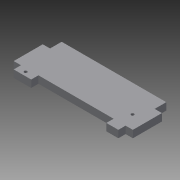
# Autodesk Inventor part: print-head-fix
Saved by Autodesk Inventor 2014 (Build 180170000, 170)
## iProperties
Created: 2014-03-01
Part Number: print-head-fix
Material: 常规
Document SubType Name: Modeling
Designer: Keshuai
Density: 1 g/cm^3
Appearance: 默认
Author: Keshuai
Autodesk Inventor part; units mm, degrees
ref_plane "YZ Plane" through (0, 0, 0) normal (1, 0, 0) x (0, 1, 0)
ref_plane "XZ Plane" through (0, 0, 0) normal (0, 1, 0) x (-1, 0, 0)
ref_plane "XY Plane" through (0, 0, 0) normal (0, 0, 1) x (1, 0, 0)
sketch "草图1" plane through (0, 0, 0) normal (0, 0, 1) x (1, 0, 0)
  line L0 (0, 0) -> (72, 0)
  line L1 (72, 0) -> (72, -33)
  line L2 (72, -33) -> (0, -33)
  line L3 (0, -33) -> (0, 0)
  line L4 (36, 26.4753) -> (36, -41.1536) construction
  line L5 (0.9, -33) -> (71.1, -33) construction
  line L6 (71.1, -33) -> (71.1, 0) construction
  line L7 (71.1, 0) -> (0.9, 0) construction
  line L8 (0.9, 0) -> (0.9, -33) construction
  line L9 (0.9, -33) -> (71.1, 0) construction
  line L10 (71.1, -33) -> (0.9, 0) construction
  circle A0 centre (5.5, -18.9) radius 1 construction
  circle A1 centre (67.7, -18.9) radius 0.75
  circle A2 centre (5.5, -30.3) radius 0.75
  line L11 (0, -8) -> (-5, -8)
  line L12 (-5, -8) -> (-5, -28)
  line L13 (-5, -28) -> (0, -28)
  line L14 (0, -28) -> (0, -8)
  line L15 (72, -8) -> (77, -8)
  line L16 (77, -8) -> (77, -28)
  line L17 (77, -28) -> (72, -28)
  line L18 (72, -28) -> (72, -8)
  point P0 (36, -16.5)
  dimension "d0" = 72
  dimension "d1" = 70.2
  dimension "d2" = 33
  dimension "d3" = 0
  dimension "d4" = 0
  dimension "d5" = 2
  dimension "d6" = 18.9
  dimension "d7" = 4.6
  dimension "d8" = 1.5
  dimension "d9" = 62.2
  dimension "d10" = 1.5
  dimension "d11" = 11.4
  dimension "d12" = 5
  dimension "d13" = 20
  dimension "d14" = 5
  dimension "d15" = 5
  dimension "d16" = 20
  dimension "d17" = 5
  constraints: 38 end point, 9 parallel, 4 horizontal, 4 perpendicular, 3 centre point, 3 point on line, 2 midpoint
  measures "d0" distance of L1.end L2.end
  measures "d1" distance of L7.end L6.end
  measures "d2" distance of L6.end L5.end
  measures "d3" distance between parallel lines of L0 L7
  measures "d4" distance between parallel lines of L2 L5
  measures "d5" diameter of A0
  measures "d6" distance from line of L7 A0.centre
  measures "d7" distance from line of L8 A0.centre
  measures "d8" diameter of A1
  measures "d9" distance of A1.centre A0.centre
  measures "d10" diameter of A2
  measures "d11" distance of A2.centre A0.centre
  measures "d12" distance of L13.end L12.end
  measures "d13" distance of L12.end L11.end
  measures "d14" distance between parallel lines of L5 L13
  measures "d15" distance of L16.end L17.end
  measures "d16" distance of L15.end L16.end
  measures "d17" distance between parallel lines of L5 L17
extrude "拉伸1" add sketch "草图1" along normal blind 5
sketch "草图2" plane through (0, 0, 5) normal (0, 0, 1) x (1, 0, 0)
  circle A0 centre (67.7, -18.9) radius 0.75 projected
  line L0 (0, -33) -> (72, -33) projected
  line L1 (72, -33) -> (72, -28) projected
  line L2 (-25.3854, -5.8) -> (85.4297, -5.8) construction
  line L3 (12.0239, -33) -> (63.7473, -33)
  line L4 (63.7473, -33) -> (63.7473, -28)
  line L5 (63.7473, -28) -> (12.0239, -28)
  line L6 (12.0239, -28) -> (12.0239, -33)
  dimension "d20" = 13.1
  constraints: 10 end point, 2 parallel, 2 perpendicular, 1 horizontal, 1 point on line
  measures "d20" distance from line of A0.centre L2
extrude "拉伸2" cut sketch "草图2" against normal through all contours L6 L5 L4 L0
